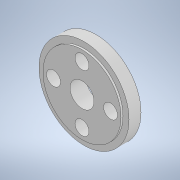
# Autodesk Inventor part: Pulley
Saved by Autodesk Inventor 2022 (Build 260153000, 153)
## iProperties
Created: 2022-08-17
Part Number: Pulley
Material: Generic
Document SubType Name: Modeling
Designer: Nick
Density: 1 g/cm^3
Appearance: Default
Author: Nick
Autodesk Inventor part; units mm, degrees
ref_plane "YZ Plane" through (0, 0, 0) normal (1, 0, 0) x (0, 1, 0)
ref_plane "XZ Plane" through (0, 0, 0) normal (0, 1, 0) x (-1, 0, 0)
ref_plane "XY Plane" through (0, 0, 0) normal (0, 0, 1) x (1, 0, 0)
sketch "Sketch1" plane through (0, 0, 0) normal (0, 0, 1) x (1, 0, 0)
  circle A0 centre (0, 0) radius 6
  circle A1 centre (0, 0) radius 22.5
  dimension "d0" = 12
  dimension "d1" = 45
  constraints: 2 centre point, 2 coincident
  measures "d0" diameter of A0
  measures "d1" diameter of A1
extrude "Extrusion1" add sketch "Sketch1" along normal blind 8
sketch "Sketch2" plane through (0, 0, 8) normal (0, 0, 1) x (1, 0, 0)
  circle A0 centre (0, 0) radius 22.5 projected
  circle A1 centre (0, 0) radius 6 projected
  circle A2 centre (0, 0) radius 6 projected
  line L0 (0, 6) -> (0, 22.5) construction
  circle A3 centre (0, 0) radius 22.5 projected
  point P0 (0, 14.25)
  point P1 (0, 14.25)
  constraints: 3 vertical alignment, 2 end point, 1 coincident, 1 midpoint, 2 other
hole "Hole1" at (0, 14.25, 8) direction (0, 0, -1) diameter 7 end through all clearance for "Flat Head Machine Screw" size "M6" standard "Ansi Metric M Profile"
pattern_circular "Circular Pattern1" count 4 over 360 about axis through (0, 0, 0) along (0, 0, 1) of "Hole1"
sketch "Sketch3" plane through (0, 0, 8) normal (0, 0, 1) x (1, 0, 0)
  circle A0 centre (14.25, 0) radius 3.5 projected
  circle A1 centre (0, -14.25) radius 3.5 projected
  circle A2 centre (-14.25, 0) radius 3.5 projected
  circle A3 centre (0, 14.25) radius 3.5 projected
  circle A4 centre (0, 0) radius 22.5 projected
  circle A5 centre (0, 0) radius 6 projected
  circle A6 centre (0, 0) radius 19.5
  dimension "d14" = 3
  constraints: 1 centre point
  measures "d14" radial gap between concentric circles of A4 A6
extrude "Extrusion2" cut sketch "Sketch3" against normal blind 1 contours A4
ref_plane "Work Plane1" through (0, 0, 4) normal (0, 0, 1) x (1, 0, 0)
mirror "Mirror1" about plane through (0, 0, 4) normal (0, 0, 1) of "Extrusion2"
body "Solid1"
